Autodesk Inventor part; units mm, degrees
(part 2 of 3)
  line L290 (55.8844, 21.002) -> (55.8694, 21.0241) construction
  line L291 (55.8694, 21.0241) -> (55.8552, 21.0458) construction
  spline S93 degree 3 poles (55.8552, 21.0458) (55.8532, 21.0498) (55.8502, 21.0528) (55.8482, 21.0569) knots 0 0 0 0 1 1 1 1
  line L292 (55.8552, 21.0458) -> (55.8532, 21.0498) construction
  line L293 (55.8532, 21.0498) -> (55.8502, 21.0528) construction
  line L294 (55.8502, 21.0528) -> (55.8482, 21.0569) construction
  spline S94 degree 3 poles (55.8482, 21.0569) (55.8363, 21.0778) (55.8253, 21.0987) (55.8154, 21.1204) knots 0 0 0 0 1 1 1 1
  line L295 (55.8482, 21.0569) -> (55.8363, 21.0778) construction
  line L296 (55.8363, 21.0778) -> (55.8253, 21.0987) construction
  line L297 (55.8253, 21.0987) -> (55.8154, 21.1204) construction
  spline S95 degree 3 poles (55.8154, 21.1204) (55.8134, 21.1244) (55.8114, 21.1274) (55.8084, 21.1314) knots 0 0 0 0 1 1 1 1
  line L298 (55.8154, 21.1204) -> (55.8134, 21.1244) construction
  line L299 (55.8134, 21.1244) -> (55.8114, 21.1274) construction
  line L300 (55.8114, 21.1274) -> (55.8084, 21.1314) construction
  spline S96 degree 3 poles (55.8084, 21.1314) (55.7984, 21.1563) (55.7887, 21.1827) (55.782, 21.2079) knots 0 0 0 0 1 1 1 1
  line L301 (55.8084, 21.1314) -> (55.7984, 21.1563) construction
  line L302 (55.7984, 21.1563) -> (55.7887, 21.1827) construction
  line L303 (55.7887, 21.1827) -> (55.782, 21.2079) construction
  spline S97 degree 3 poles (55.782, 21.2079) (55.781, 21.2109) (55.78, 21.2149) (55.779, 21.2182) knots 0 0 0 0 1 1 1 1
  line L304 (55.782, 21.2079) -> (55.781, 21.2109) construction
  line L305 (55.781, 21.2109) -> (55.78, 21.2149) construction
  line L306 (55.78, 21.2149) -> (55.779, 21.2182) construction
  spline S98 degree 3 poles (55.779, 21.2182) (55.773, 21.2411) (55.7679, 21.264) (55.7652, 21.2865) knots 0 0 0 0 1 1 1 1
  line L307 (55.779, 21.2182) -> (55.773, 21.2411) construction
  line L308 (55.773, 21.2411) -> (55.7679, 21.264) construction
  line L309 (55.7679, 21.264) -> (55.7652, 21.2865) construction
  spline S99 degree 3 poles (55.7652, 21.2865) (55.7642, 21.2935) (55.7632, 21.2999) (55.7612, 21.3058) knots 0 0 0 0 1 1 1 1
  line L310 (55.7652, 21.2865) -> (55.7642, 21.2935) construction
  line L311 (55.7642, 21.2935) -> (55.7632, 21.2999) construction
  line L312 (55.7632, 21.2999) -> (55.7612, 21.3058) construction
  spline S100 degree 3 poles (55.7612, 21.3058) (55.7582, 21.333) (55.7552, 21.3595) (55.7552, 21.3863) knots 0 0 0 0 1 1 1 1
  line L313 (55.7612, 21.3058) -> (55.7582, 21.333) construction
  line L314 (55.7582, 21.333) -> (55.7552, 21.3595) construction
  line L315 (55.7552, 21.3595) -> (55.7552, 21.3863) construction
  spline S101 degree 3 poles (55.7552, 21.3863) (54.9688, 22.0101) (54.9511, 22.0101) (54.9511, 22.0101) knots 0 0 0 0 1 1 1 1
  line L316 (55.7552, 21.3863) -> (54.9688, 22.0101) construction
  line L317 (54.9688, 22.0101) -> (54.9511, 22.0101) construction
  line L318 (54.9511, 22.0101) -> (54.9511, 22.0101) construction
  line L319 (56.1953, 20.7863) -> (56.1903, 20.7883)
  spline S102 degree 3 poles (56.3621, 22.0101) (56.3747, 22.0101) (56.3877, 22.0101) (56.4012, 22.0097) knots 0 0 0 0 1 1 1 1
  line L320 (56.3621, 22.0101) -> (56.3747, 22.0101) construction
  line L321 (56.3747, 22.0101) -> (56.3877, 22.0101) construction
  line L322 (56.3877, 22.0101) -> (56.4012, 22.0097) construction
  spline S103 degree 3 poles (56.4012, 22.0097) (57.2626, 21.9765) (57.984, 20.9159) (58.8359, 20.7624) knots 0 0 0 0 1 1 1 1
  line L323 (56.4012, 22.0097) -> (57.2626, 21.9765) construction
  line L324 (57.2626, 21.9765) -> (57.984, 20.9159) construction
  line L325 (57.984, 20.9159) -> (58.8359, 20.7624) construction
  spline S104 degree 3 poles (58.8359, 20.7624) (58.5092, 20.7624) (57.8822, 20.5998) (56.9505, 21.2379) knots 0 0 0 0 1 1 1 1
  line L326 (58.8359, 20.7624) -> (58.5092, 20.7624) construction
  line L327 (58.5092, 20.7624) -> (57.8822, 20.5998) construction
  line L328 (57.8822, 20.5998) -> (56.9505, 21.2379) construction
  line L329 (54.9511, 22.0101) -> (56.3621, 22.0101)
  spline S105 degree 3 poles (56.3625, 21.7778) (56.3625, 21.7776) (56.3136, 21.6503) (56.2426, 21.554) knots 0 0 0 0 1 1 1 1
  line L330 (56.3625, 21.7778) -> (56.3625, 21.7778) construction
  line L331 (56.3625, 21.7778) -> (56.3136, 21.6503) construction
  line L332 (56.3136, 21.6503) -> (56.2426, 21.554) construction
  spline S106 degree 3 poles (56.2426, 21.554) (56.2055, 21.5027) (56.1601, 21.4546) (56.1601, 21.3863) knots 0 0 0 0 1 1 1 1
  line L333 (56.2426, 21.554) -> (56.2055, 21.5027) construction
  line L334 (56.2055, 21.5027) -> (56.1601, 21.4546) construction
  line L335 (56.1601, 21.4546) -> (56.1601, 21.3863) construction
  spline S107 degree 3 poles (56.1601, 21.3863) (56.1601, 21.318) (56.2047, 21.2699) (56.2422, 21.219) knots 0 0 0 0 1 1 1 1
  line L336 (56.1601, 21.3863) -> (56.1601, 21.318) construction
  line L337 (56.1601, 21.318) -> (56.2047, 21.2699) construction
  line L338 (56.2047, 21.2699) -> (56.2422, 21.219) construction
  spline S108 degree 3 poles (56.2422, 21.219) (56.3128, 21.1215) (56.3625, 20.9946) (56.3625, 20.9945) knots 0 0 0 0 1 1 1 1
  line L339 (56.2422, 21.219) -> (56.3128, 21.1215) construction
  line L340 (56.3128, 21.1215) -> (56.3625, 20.9945) construction
  line L341 (56.3625, 20.9945) -> (56.3625, 20.9945) construction
  spline S109 degree 3 poles (56.3625, 20.9945) (56.3626, 20.9946) (56.411, 21.1216) (56.4821, 21.2186) knots 0 0 0 0 1 1 1 1
  line L342 (56.3625, 20.9945) -> (56.3625, 20.9945) construction
  line L343 (56.3625, 20.9945) -> (56.411, 21.1216) construction
  line L344 (56.411, 21.1216) -> (56.4821, 21.2186) construction
  spline S110 degree 3 poles (56.4821, 21.2186) (56.5192, 21.2695) (56.5642, 21.3176) (56.5642, 21.3863) knots 0 0 0 0 1 1 1 1
  line L345 (56.4821, 21.2186) -> (56.5192, 21.2695) construction
  line L346 (56.5192, 21.2695) -> (56.5642, 21.3176) construction
  line L347 (56.5642, 21.3176) -> (56.5642, 21.3863) construction
  spline S111 degree 3 poles (56.5642, 21.3863) (56.5642, 21.455) (56.52, 21.5023) (56.4825, 21.5532) knots 0 0 0 0 1 1 1 1
  line L348 (56.5642, 21.3863) -> (56.5642, 21.455) construction
  line L349 (56.5642, 21.455) -> (56.52, 21.5023) construction
  line L350 (56.52, 21.5023) -> (56.4825, 21.5532) construction
  spline S112 degree 3 poles (56.4825, 21.5532) (56.4119, 21.6503) (56.3625, 21.7778) (56.3625, 21.7778) knots 0 0 0 0 1 1 1 1
  line L351 (56.4825, 21.5532) -> (56.4119, 21.6503) construction
  line L352 (56.4119, 21.6503) -> (56.3625, 21.7778) construction
  line L353 (56.3625, 21.7778) -> (56.3625, 21.7778) construction
  line L354 (56.9505, 21.2379) -> (56.9513, 21.2376)
  spline S113 degree 3 poles (56.4825, 21.5532) (56.4119, 21.6503) (56.3626, 21.7776) (56.3625, 21.7778) knots 0 0 0 0 1 1 1 1
  line L355 (56.4825, 21.5532) -> (56.4119, 21.6503) construction
  line L356 (56.4119, 21.6503) -> (56.3625, 21.7778) construction
  line L357 (56.3625, 21.7778) -> (56.3625, 21.7778) construction
  spline S114 degree 3 poles (56.3625, 21.7778) (56.3625, 21.7776) (56.3136, 21.6503) (56.2426, 21.554) knots 0 0 0 0 1 1 1 1
  line L358 (56.3625, 21.7778) -> (56.3625, 21.7778) construction
  line L359 (56.3625, 21.7778) -> (56.3136, 21.6503) construction
  line L360 (56.3136, 21.6503) -> (56.2426, 21.554) construction
  spline S115 degree 3 poles (56.2426, 21.554) (56.2055, 21.5027) (56.1601, 21.4546) (56.1601, 21.3863) knots 0 0 0 0 1 1 1 1
  line L361 (56.2426, 21.554) -> (56.2055, 21.5027) construction
  line L362 (56.2055, 21.5027) -> (56.1601, 21.4546) construction
  line L363 (56.1601, 21.4546) -> (56.1601, 21.3863) construction
  spline S116 degree 3 poles (56.1601, 21.3863) (56.1601, 21.318) (56.2047, 21.2699) (56.2422, 21.219) knots 0 0 0 0 1 1 1 1
  line L364 (56.1601, 21.3863) -> (56.1601, 21.318) construction
  line L365 (56.1601, 21.318) -> (56.2047, 21.2699) construction
  line L366 (56.2047, 21.2699) -> (56.2422, 21.219) construction
  spline S117 degree 3 poles (56.2422, 21.219) (56.3128, 21.1215) (56.3625, 20.9946) (56.3625, 20.9945) knots 0 0 0 0 1 1 1 1
  line L367 (56.2422, 21.219) -> (56.3128, 21.1215) construction
  line L368 (56.3128, 21.1215) -> (56.3625, 20.9945) construction
  line L369 (56.3625, 20.9945) -> (56.3625, 20.9945) construction
  spline S118 degree 3 poles (56.3625, 20.9945) (56.3626, 20.9946) (56.411, 21.1216) (56.4821, 21.2186) knots 0 0 0 0 1 1 1 1
  line L370 (56.3625, 20.9945) -> (56.3625, 20.9945) construction
  line L371 (56.3625, 20.9945) -> (56.411, 21.1216) construction
  line L372 (56.411, 21.1216) -> (56.4821, 21.2186) construction
  spline S119 degree 3 poles (56.4821, 21.2186) (56.5192, 21.2695) (56.5642, 21.3176) (56.5642, 21.3863) knots 0 0 0 0 1 1 1 1
  line L373 (56.4821, 21.2186) -> (56.5192, 21.2695) construction
  line L374 (56.5192, 21.2695) -> (56.5642, 21.3176) construction
  line L375 (56.5642, 21.3176) -> (56.5642, 21.3863) construction
  spline S120 degree 3 poles (56.5642, 21.3863) (56.5642, 21.455) (56.52, 21.5023) (56.4825, 21.5532) knots 0 0 0 0 1 1 1 1
  line L376 (56.5642, 21.3863) -> (56.5642, 21.455) construction
  line L377 (56.5642, 21.455) -> (56.52, 21.5023) construction
  line L378 (56.52, 21.5023) -> (56.4825, 21.5532) construction
  spline S121 degree 3 poles (62.9834, 11.6734) (62.6228, 13.9494) (60.8593, 15.3143) (55.8176, 16.2629) knots 0 0 0 0 1 1 1 1
  line L379 (62.9834, 11.6734) -> (62.6228, 13.9494) construction
  line L380 (62.6228, 13.9494) -> (60.8593, 15.3143) construction
  line L381 (60.8593, 15.3143) -> (55.8176, 16.2629) construction
  spline S122 degree 3 poles (55.8176, 16.2629) (54.8047, 16.4322) (54.6007, 17.116) (54.9542, 17.6791) knots 0 0 0 0 1 1 1 1
  line L382 (55.8176, 16.2629) -> (54.8047, 16.4322) construction
  line L383 (54.8047, 16.4322) -> (54.6007, 17.116) construction
  line L384 (54.6007, 17.116) -> (54.9542, 17.6791) construction
  spline S123 degree 3 poles (54.9542, 17.6791) (54.5048, 17.9459) (54.1315, 18.2363) (53.8782, 18.7418) knots 0 0 0 0 1 1 1 1
  line L385 (54.9542, 17.6791) -> (54.5048, 17.9459) construction
  line L386 (54.5048, 17.9459) -> (54.1315, 18.2363) construction
  line L387 (54.1315, 18.2363) -> (53.8782, 18.7418) construction
  spline S124 degree 3 poles (53.8782, 18.7418) (52.7216, 17.2451) (52.3416, 14.941) (53.1048, 13.0623) knots 0 0 0 0 1 1 1 1
  line L388 (53.8782, 18.7418) -> (52.7216, 17.2451) construction
  line L389 (52.7216, 17.2451) -> (52.3416, 14.941) construction
  line L390 (52.3416, 14.941) -> (53.1048, 13.0623) construction
  spline S125 degree 3 poles (53.1048, 13.0623) (53.1348, 13.9518) (53.525, 14.653) (54.1374, 14.9501) knots 0 0 0 0 1 1 1 1
  line L391 (53.1048, 13.0623) -> (53.1348, 13.9518) construction
  line L392 (53.1348, 13.9518) -> (53.525, 14.653) construction
  line L393 (53.525, 14.653) -> (54.1374, 14.9501) construction
  spline S126 degree 3 poles (54.1374, 14.9501) (55.0797, 15.4074) (56.4442, 15.1123) (56.5535, 14.9331) knots 0 0 0 0 1 1 1 1
  line L394 (54.1374, 14.9501) -> (55.0797, 15.4074) construction
  line L395 (55.0797, 15.4074) -> (56.4442, 15.1123) construction
  line L396 (56.4442, 15.1123) -> (56.5535, 14.9331) construction
  spline S127 degree 3 poles (56.5535, 14.9331) (55.8089, 14.8514) (55.204, 14.9371) (54.4294, 14.4249) knots 0 0 0 0 1 1 1 1
  line L397 (56.5535, 14.9331) -> (55.8089, 14.8514) construction
  line L398 (55.8089, 14.8514) -> (55.204, 14.9371) construction
  line L399 (55.204, 14.9371) -> (54.4294, 14.4249) construction
  spline S128 degree 3 poles (54.4294, 14.4249) (52.6506, 12.7652) (54.459, 11.7728) (54.7214, 11.0889) knots 0 0 0 0 1 1 1 1
  line L400 (54.4294, 14.4249) -> (52.6506, 12.7652) construction
  line L401 (52.6506, 12.7652) -> (54.459, 11.7728) construction
  line L402 (54.459, 11.7728) -> (54.7214, 11.0889) construction
  spline S129 degree 3 poles (51.5856, 11.3809) (51.0442, 10.6983) (50.6141, 10.0602) (50.4077, 9.5121) knots 0 0 0 0 1 1 1 1
  line L403 (51.5856, 11.3809) -> (51.0442, 10.6983) construction
  line L404 (51.0442, 10.6983) -> (50.6141, 10.0602) construction
  line L405 (50.6141, 10.0602) -> (50.4077, 9.5121) construction
  spline S130 degree 3 poles (50.4077, 9.5121) (50.5142, 8.7466) (50.8303, 8.2471) (51.3737, 8.032) knots 0 0 0 0 1 1 1 1
  line L406 (50.4077, 9.5121) -> (50.5142, 8.7466) construction
  line L407 (50.5142, 8.7466) -> (50.8303, 8.2471) construction
  line L408 (50.8303, 8.2471) -> (51.3737, 8.032) construction
  line L409 (54.7214, 11.0889) -> (51.5856, 11.3809)
  spline S131 degree 3 poles (51.4565, 8.4105) (51.2667, 8.7786) (51.1629, 9.1022) (51.1764, 9.3638) knots 0 0 0 0 1 1 1 1
  line L410 (51.4565, 8.4105) -> (51.2667, 8.7786) construction
  line L411 (51.2667, 8.7786) -> (51.1629, 9.1022) construction
  line L412 (51.1629, 9.1022) -> (51.1764, 9.3638) construction
  spline S132 degree 3 poles (51.1764, 9.3638) (51.3401, 9.7774) (51.6163, 10.1601) (51.9916, 10.5156) knots 0 0 0 0 1 1 1 1
  line L413 (51.1764, 9.3638) -> (51.3401, 9.7774) construction
  line L414 (51.3401, 9.7774) -> (51.6163, 10.1601) construction
  line L415 (51.6163, 10.1601) -> (51.9916, 10.5156) construction
  spline S133 degree 3 poles (51.9916, 10.5156) (52.9611, 10.1356) (54.0131, 9.8022) (55.1535, 9.5173) knots 0 0 0 0 1 1 1 1
  line L416 (51.9916, 10.5156) -> (52.9611, 10.1356) construction
  line L417 (52.9611, 10.1356) -> (54.0131, 9.8022) construction
  line L418 (54.0131, 9.8022) -> (55.1535, 9.5173) construction
  line L419 (51.3737, 8.032) -> (51.9435, 7.9914)
  line L420 (51.9435, 7.9914) -> (51.4565, 8.4105)
  spline S134 degree 3 poles (55.9166, 9.8571) (56.1155, 9.9518) (56.2978, 10.0437) (56.471, 10.1345) knots 0 0 0 0 1 1 1 1
  line L421 (55.9166, 9.8571) -> (56.1155, 9.9518) construction
  line L422 (56.1155, 9.9518) -> (56.2978, 10.0437) construction
  line L423 (56.2978, 10.0437) -> (56.471, 10.1345) construction
  line L424 (55.1535, 9.5173) -> (55.4226, 9.6373)
  line L425 (55.4226, 9.6373) -> (55.9166, 9.8571)
  spline S135 degree 3 poles (55.5457, 12.5088) (55.419, 12.7992) (55.3756, 13.0442) (55.6025, 13.1393) knots 0 0 0 0 1 1 1 1
  line L426 (55.5457, 12.5088) -> (55.419, 12.7992) construction
  line L427 (55.419, 12.7992) -> (55.3756, 13.0442) construction
  line L428 (55.3756, 13.0442) -> (55.6025, 13.1393) construction
  spline S136 degree 3 poles (55.6025, 13.1393) (56.2031, 13.1463) (56.9923, 12.9038) (57.0451, 12.8868) knots 0 0 0 0 1 1 1 1
  line L429 (55.6025, 13.1393) -> (56.2031, 13.1463) construction
  line L430 (56.2031, 13.1463) -> (56.9923, 12.9038) construction
  line L431 (56.9923, 12.9038) -> (57.0451, 12.8868) construction
  spline S137 degree 3 poles (57.0451, 12.8868) (57.0119, 12.8928) (56.6687, 12.9484) (56.0847, 12.7491) knots 0 0 0 0 1 1 1 1
  line L432 (57.0451, 12.8868) -> (57.0119, 12.8928) construction
  line L433 (57.0119, 12.8928) -> (56.6687, 12.9484) construction
  line L434 (56.6687, 12.9484) -> (56.0847, 12.7491) construction
  line L435 (56.471, 10.1345) -> (56.4552, 10.1728)
  line L436 (56.4552, 10.1728) -> (55.5457, 12.5088)
  spline S138 degree 3 poles (57.2353, 10.5733) (58.8015, 11.5763) (58.8832, 12.3995) (58.7486, 13.2656) knots 0 0 0 0 1 1 1 1
  line L437 (57.2353, 10.5733) -> (58.8015, 11.5763) construction
  line L438 (58.8015, 11.5763) -> (58.8832, 12.3995) construction
  line L439 (58.8832, 12.3995) -> (58.7486, 13.2656) construction
  spline S139 degree 3 poles (58.7486, 13.2656) (58.6819, 13.6945) (58.5655, 14.1144) (58.4025, 14.5149) knots 0 0 0 0 1 1 1 1
  line L440 (58.7486, 13.2656) -> (58.6819, 13.6945) construction
  line L441 (58.6819, 13.6945) -> (58.5655, 14.1144) construction
  line L442 (58.5655, 14.1144) -> (58.4025, 14.5149) construction
  spline S140 degree 3 poles (58.4025, 14.5149) (58.8883, 14.3949) (59.3393, 14.1554) (59.7154, 13.8161) knots 0 0 0 0 1 1 1 1
  line L443 (58.4025, 14.5149) -> (58.8883, 14.3949) construction
  line L444 (58.8883, 14.3949) -> (59.3393, 14.1554) construction
  line L445 (59.3393, 14.1554) -> (59.7154, 13.8161) construction
  spline S141 degree 3 poles (59.7154, 13.8161) (61.8793, 11.8644) (63.5682, 4.8248) (54.0229, 2.8183) knots 0 0 0 0 1 1 1 1
  line L446 (59.7154, 13.8161) -> (61.8793, 11.8644) construction
  line L447 (61.8793, 11.8644) -> (63.5682, 4.8248) construction
  line L448 (63.5682, 4.8248) -> (54.0229, 2.8183) construction
  line L449 (56.0847, 12.7491) -> (57.2353, 10.5733)
  spline S142 degree 3 poles (54.0299, 2.8183) (58.7114, 3.0811) (63.9958, 5.2928) (62.9833, 11.6734) knots 0 0 0 0 1 1 1 1
  line L450 (54.0299, 2.8183) -> (58.7114, 3.0811) construction
  line L451 (58.7114, 3.0811) -> (63.9958, 5.2928) construction
  line L452 (63.9958, 5.2928) -> (62.9833, 11.6734) construction
  line L453 (54.0229, 2.8183) -> (54.0299, 2.8183)
  line L454 (62.9833, 11.6734) -> (62.9834, 11.6734)
  point P0 (0, 0)
  constraints: 52 end point, 429 other
sketch "Szkic14" plane through (0, 0, 2.5) normal (0, 0, 1) x (1, 0, 0)
  line L0 (-6.6512, 10.9422) -> (-6.5928, 10.8137) construction
  line L1 (-6.5928, 10.8137) -> (-6.4673, 10.6328) construction
  line L2 (-6.4673, 10.6328) -> (-6.3389, 10.4489) construction
  line L3 (-6.3389, 10.4489) -> (-6.0849, 10.1628) construction
  line L4 (-6.0849, 10.1628) -> (-5.8893, 9.9935) construction
  line L5 (-5.8893, 9.9935) -> (-5.6704, 9.8271) construction
  line L6 (-5.6704, 9.8271) -> (-5.4544, 9.687) construction
  line L7 (-5.4544, 9.687) -> (-5.2589, 9.5674) construction
  spline S0 degree 4 poles (-6.6512, 10.9422) (-6.5928, 10.8137) (-6.4673, 10.6328) (-6.3389, 10.4489) (-6.0849, 10.1628) (-5.8893, 9.9935) (-5.6704, 9.8271) (-5.4544, 9.687) (-5.2589, 9.5674) knots 1 1 1 1 1 2 3 4 5 6 6 6 6 6
  line L8 (-5.2589, 9.5674) -> (-5.4035, 9.331) construction
  line L9 (-5.4035, 9.331) -> (-5.4544, 9.0682) construction
  line L10 (-5.4544, 9.0682) -> (-5.4544, 8.9077) construction
  line L11 (-5.4544, 8.9077) -> (-5.4544, 8.7325) construction
  line L12 (-5.4544, 8.7325) -> (-5.4106, 8.5574) construction
  line L13 (-5.4106, 8.5574) -> (-5.3378, 8.3971) construction
  line L14 (-5.3378, 8.3971) -> (-5.2384, 8.2538) construction
  line L15 (-5.2384, 8.2538) -> (-5.0652, 8.1039) construction
  line L16 (-5.0652, 8.1039) -> (-4.9181, 7.9921) construction
  line L17 (-4.9181, 7.9921) -> (-4.7393, 7.8984) construction
  line L18 (-4.7393, 7.8984) -> (-4.596, 7.8481) construction
  line L19 (-4.596, 7.8481) -> (-4.3639, 7.7777) construction
  line L20 (-4.3639, 7.7777) -> (-4.0614, 7.7125) construction
  line L21 (-4.0614, 7.7125) -> (-3.7401, 7.6548) construction
  line L22 (-3.7401, 7.6548) -> (-3.2763, 7.5488) construction
  line L23 (-3.2763, 7.5488) -> (-2.8258, 7.4561) construction
  spline S1 degree 4 poles (-5.2589, 9.5674) (-5.4035, 9.331) (-5.4544, 9.0682) (-5.4544, 8.9077) (-5.4544, 8.7325) (-5.4106, 8.5574) (-5.3378, 8.3971) (-5.2384, 8.2538) (-5.0652, 8.1039) (-4.9181, 7.9921) (-4.7393, 7.8984) (-4.596, 7.8481) (-4.3639, 7.7777) (-4.0614, 7.7125) (-3.7401, 7.6548) (-3.2763, 7.5488) (-2.8258, 7.4561) knots 1 1 1 1 1 2 3 4 5 6 7 8 9 10 11 12 13 14 14 14 14 14
  line L24 (-2.8258, 7.4561) -> (-2.2142, 7.3144) construction
  line L25 (-2.2142, 7.3144) -> (-1.5745, 7.1703) construction
  line L26 (-1.5745, 7.1703) -> (-0.9584, 6.9834) construction
  line L27 (-0.9584, 6.9834) -> (-0.2587, 6.7712) construction
  line L28 (-0.2587, 6.7712) -> (0.4179, 6.5333) construction
  line L29 (0.4179, 6.5333) -> (1.2289, 6.2149) construction
  line L30 (1.2289, 6.2149) -> (1.8914, 5.9102) construction
  line L31 (1.8914, 5.9102) -> (2.8245, 5.3392) construction
  line L32 (2.8245, 5.3392) -> (3.3345, 4.9516) construction
  line L33 (3.3345, 4.9516) -> (3.839, 4.4666) construction
  line L34 (3.839, 4.4666) -> (4.1432, 4.1239) construction
  line L35 (4.1432, 4.1239) -> (4.4557, 3.6733) construction
  line L36 (4.4557, 3.6733) -> (4.6713, 3.2438) construction
  line L37 (4.6713, 3.2438) -> (4.8704, 2.8057) construction
  line L38 (4.8704, 2.8057) -> (4.945, 2.5074) construction
  line L39 (4.945, 2.5074) -> (5.0688, 2.0124) construction
  line L40 (5.0688, 2.0124) -> (5.1432, 1.5744) construction
  line L41 (5.1432, 1.5744) -> (5.1888, 0.9732) construction
  line L42 (5.1888, 0.9732) -> (5.2151, 0.3807) construction
  line L43 (5.2151, 0.3807) -> (5.2602, -0.5324) construction
  line L44 (5.2602, -0.5324) -> (5.1507, -1.5377) construction
  line L45 (5.1507, -1.5377) -> (4.9589, -2.5271) construction
  line L46 (4.9589, -2.5271) -> (4.707, -3.3577) construction
  line L47 (4.707, -3.3577) -> (4.6129, -3.6252) construction
  line L48 (4.6129, -3.6252) -> (4.4152, -4.0747) construction
  line L49 (4.4152, -4.0747) -> (3.746, -5.2202) construction
  line L50 (3.746, -5.2202) -> (3.0018, -6.0798) construction
  line L51 (3.0018, -6.0798) -> (2.3815, -6.6305) construction
  line L52 (2.3815, -6.6305) -> (1.6684, -7.2033) construction
  line L53 (1.6684, -7.2033) -> (0.6461, -7.8274) construction
  line L54 (0.6461, -7.8274) -> (-0.713, -8.472) construction
  line L55 (-0.713, -8.472) -> (-2.0638, -8.9236) construction
  line L56 (-2.0638, -8.9236) -> (-3.5466, -9.2943) construction
  line L57 (-3.5466, -9.2943) -> (-5.0652, -9.5408) construction
  line L58 (-5.0652, -9.5408) -> (-6.4673, -9.6692) construction
  spline S2 degree 4 poles (-2.8258, 7.4561) (-2.2142, 7.3144) (-1.5745, 7.1703) (-0.9584, 6.9834) (-0.2587, 6.7712) (0.4179, 6.5333) (1.2289, 6.2149) (1.8914, 5.9102) (2.8245, 5.3392) (3.3345, 4.9516) (3.839, 4.4666) (4.1432, 4.1239) (4.4557, 3.6733) (4.6713, 3.2438) (4.8704, 2.8057) (4.945, 2.5074) (5.0688, 2.0124) (5.1432, 1.5744) (5.1888, 0.9732) (5.2151, 0.3807) (5.2602, -0.5324) (5.1507, -1.5377) (4.9589, -2.5271) (4.707, -3.3577) (4.6129, -3.6252) (4.4152, -4.0747) (3.746, -5.2202) (3.0018, -6.0798) (2.3815, -6.6305) (1.6684, -7.2033) (0.6461, -7.8274) (-0.713, -8.472) (-2.0638, -8.9236) (-3.5466, -9.2943) (-5.0652, -9.5408) (-6.4673, -9.6692) knots 1 1 1 1 1 2 3 4 5 6 7 8 9 10 11 12 13 14 15 16 17 18 19 20 21 22 23 24 25 26 27 28 29 30 31 32 33 33 33 33 33
  line L59 (-6.4673, -9.6692) -> (-4.596, -9.174) construction
  line L60 (-4.596, -9.174) -> (-3.6929, -8.872) construction
  line L61 (-3.6929, -8.872) -> (-2.1422, -8.2833) construction
  line L62 (-2.1422, -8.2833) -> (-1.296, -7.901) construction
  line L63 (-1.296, -7.901) -> (-0.6086, -7.3619) construction
  line L64 (-0.6086, -7.3619) -> (0.1327, -6.8478) construction
  line L65 (0.1327, -6.8478) -> (0.6779, -6.2808) construction
  line L66 (0.6779, -6.2808) -> (1.3083, -5.7211) construction
  line L67 (1.3083, -5.7211) -> (1.8469, -5.0124) construction
  line L68 (1.8469, -5.0124) -> (2.3815, -4.2056) construction
  line L69 (2.3815, -4.2056) -> (2.5915, -3.6252) construction
  line L70 (2.5915, -3.6252) -> (2.7867, -2.9832) construction
  line L71 (2.7867, -2.9832) -> (2.8933, -2.4331) construction
  line L72 (2.8933, -2.4331) -> (2.9439, -2.2891) construction
  line L73 (2.9439, -2.2891) -> (3.0251, -1.8703) construction
  line L74 (3.0251, -1.8703) -> (3.0795, -1.3802) construction
  line L75 (3.0795, -1.3802) -> (3.0795, -0.9391) construction
  line L76 (3.0795, -0.9391) -> (3.0444, -0.4767) construction
  line L77 (3.0444, -0.4767) -> (3.0018, 0.0093) construction
  line L78 (3.0018, 0.0093) -> (2.9748, 0.3807) construction
  line L79 (2.9748, 0.3807) -> (2.902, 0.7996) construction
  line L80 (2.902, 0.7996) -> (2.8245, 1.096) construction
  line L81 (2.8245, 1.096) -> (2.6916, 1.5744) construction
  line L82 (2.6916, 1.5744) -> (2.5274, 2.0615) construction
  line L83 (2.5274, 2.0615) -> (2.358, 2.4623) construction
  line L84 (2.358, 2.4623) -> (2.1656, 2.8856) construction
  line L85 (2.1656, 2.8856) -> (1.8914, 3.3203) construction
  line L86 (1.8914, 3.3203) -> (1.5602, 3.796) construction
  line L87 (1.5602, 3.796) -> (1.1327, 4.2607) construction
  line L88 (1.1327, 4.2607) -> (0.6123, 4.7937) construction
  line L89 (0.6123, 4.7937) -> (-0.1776, 5.2552) construction
  line L90 (-0.1776, 5.2552) -> (-0.7923, 5.4713) construction
  spline S3 degree 4 poles (-6.4673, -9.6692) (-4.596, -9.174) (-3.6929, -8.872) (-2.1422, -8.2833) (-1.296, -7.901) (-0.6086, -7.3619) (0.1327, -6.8478) (0.6779, -6.2808) (1.3083, -5.7211) (1.8469, -5.0124) (2.3815, -4.2056) (2.5915, -3.6252) (2.7867, -2.9832) (2.8933, -2.4331) (2.9439, -2.2891) (3.0251, -1.8703) (3.0795, -1.3802) (3.0795, -0.9391) (3.0444, -0.4767) (3.0018, 0.0093) (2.9748, 0.3807) (2.902, 0.7996) (2.8245, 1.096) (2.6916, 1.5744) (2.5274, 2.0615) (2.358, 2.4623) (2.1656, 2.8856) (1.8914, 3.3203) (1.5602, 3.796) (1.1327, 4.2607) (0.6123, 4.7937) (-0.1776, 5.2552) (-0.7923, 5.4713) knots 1 1 1 1 1 2 3 4 5 6 7 8 9 10 11 12 13 14 15 16 17 18 19 20 21 22 23 24 25 26 27 28 29 30 30 30 30 30
  line L91 (-0.7923, 5.4713) -> (-0.4849, 4.5272) construction
  line L92 (-0.4849, 4.5272) -> (-0.4074, 4.1857) construction
  line L93 (-0.4074, 4.1857) -> (-0.3088, 3.605) construction
  line L94 (-0.3088, 3.605) -> (-0.2587, 3.1864) construction
  line L95 (-0.2587, 3.1864) -> (-0.3231, 2.5956) construction
  line L96 (-0.3231, 2.5956) -> (-0.6086, 2.0124) construction
  line L97 (-0.6086, 2.0124) -> (-0.9875, 1.4524) construction
  line L98 (-0.9875, 1.4524) -> (-1.296, 1.0568) construction
  line L99 (-1.296, 1.0568) -> (-1.7784, 0.7017) construction
  line L100 (-1.7784, 0.7017) -> (-2.309, 0.344) construction
  spline S4 degree 4 poles (-0.7923, 5.4713) (-0.4849, 4.5272) (-0.4074, 4.1857) (-0.3088, 3.605) (-0.2587, 3.1864) (-0.3231, 2.5956) (-0.6086, 2.0124) (-0.9875, 1.4524) (-1.296, 1.0568) (-1.7784, 0.7017) (-2.309, 0.344) knots 1 1 1 1 1 2 3 4 5 6 7 8 8 8 8 8
  line L101 (-2.309, 0.344) -> (-2.5669, 0.9223) construction
  line L102 (-2.5669, 0.9223) -> (-2.9657, 1.6305) construction
  line L103 (-2.9657, 1.6305) -> (-3.1735, 2.0877) construction
  line L104 (-3.1735, 2.0877) -> (-3.4271, 2.6566) construction
  line L105 (-3.4271, 2.6566) -> (-3.8071, 3.1864) construction
  spline S5 degree 4 poles (-2.309, 0.344) (-2.5669, 0.9223) (-2.9657, 1.6305) (-3.1735, 2.0877) (-3.4271, 2.6566) (-3.8071, 3.1864) knots 1 1 1 1 1 2 3 3 3 3 3
  line L106 (-3.8071, 3.1864) -> (-3.5082, 3.2675) construction
  line L107 (-3.5082, 3.2675) -> (-3.101, 3.3757) construction
  line L108 (-3.101, 3.3757) -> (-2.5516, 3.3626) construction
  spline S6 degree 3 poles (-3.8071, 3.1864) (-3.5082, 3.2675) (-3.101, 3.3757) (-2.5516, 3.3626) knots 1 1 1 1 2 2 2 2
  line L109 (-2.5516, 3.3626) -> (-3.6577, 3.6945) construction
  line L110 (-3.6577, 3.6945) -> (-4.4013, 3.6945) construction
  spline S7 degree 2 poles (-2.5516, 3.3626) (-3.6577, 3.6945) (-4.4013, 3.6945) knots 1 1 1 2 2 2
  line L111 (-4.4013, 3.6945) -> (-4.7094, 3.5581) construction
  line L112 (-4.7094, 3.5581) -> (-4.6553, 3.2438) construction
  line L113 (-4.6553, 3.2438) -> (-4.5019, 2.891) construction
  spline S8 degree 3 poles (-4.4013, 3.6945) (-4.7094, 3.5581) (-4.6553, 3.2438) (-4.5019, 2.891) knots 1 1 1 1 2 2 2 2
  line L114 (-4.5019, 2.891) -> (-3.2936, -0.1999) construction
  spline S9 degree 1 poles (-4.5019, 2.891) (-3.2936, -0.1999) knots 1 1 2 2
  line L115 (-3.2936, -0.1999) -> (-4.9917, -1.0028) construction
  spline S10 degree 1 poles (-3.2936, -0.1999) (-4.9917, -1.0028) knots 1 1 2 2
  line L116 (-4.9917, -1.0028) -> (-6.474, -0.6289) construction
  line L117 (-6.474, -0.6289) -> (-7.8356, -0.1999) construction
  line L118 (-7.8356, -0.1999) -> (-9.0893, 0.2923) construction
  spline S11 degree 3 poles (-4.9917, -1.0028) (-6.474, -0.6289) (-7.8356, -0.1999) (-9.0893, 0.2923) knots 1 1 1 1 2 2 2 2
  line L119 (-9.0893, 0.2923) -> (-9.5782, -0.1675) construction
  line L120 (-9.5782, -0.1675) -> (-9.9324, -0.6627) construction
  line L121 (-9.9324, -0.6627) -> (-10.1402, -1.1921) construction
  spline S12 degree 3 poles (-9.0893, 0.2923) (-9.5782, -0.1675) (-9.9324, -0.6627) (-10.1402, -1.1921) knots 1 1 1 1 2 2 2 2
  line L122 (-10.1402, -1.1921) -> (-10.1643, -1.5377) construction
  line L123 (-10.1643, -1.5377) -> (-10.0286, -1.9545) construction
  line L124 (-10.0286, -1.9545) -> (-9.7859, -2.4331) construction
  spline S13 degree 3 poles (-10.1402, -1.1921) (-10.1643, -1.5377) (-10.0286, -1.9545) (-9.7859, -2.4331) knots 1 1 1 1 2 2 2 2
  line L125 (-9.7859, -2.4331) -> (-9.159, -2.9734) construction
  spline S14 degree 1 poles (-9.7859, -2.4331) (-9.159, -2.9734) knots 1 1 2 2
  line L126 (-9.159, -2.9734) -> (-9.8893, -2.9225) construction
  spline S15 degree 1 poles (-9.159, -2.9734) (-9.8893, -2.9225) knots 1 1 2 2
  line L127 (-9.8893, -2.9225) -> (-10.5931, -2.6463) construction
  line L128 (-10.5931, -2.6463) -> (-10.9937, -1.9901) construction
  line L129 (-10.9937, -1.9901) -> (-11.1401, -1.006) construction
  spline S16 degree 3 poles (-9.8893, -2.9225) (-10.5931, -2.6463) (-10.9937, -1.9901) (-11.1401, -1.006) knots 1 1 1 1 2 2 2 2
  line L130 (-11.1401, -1.006) -> (-10.8707, -0.2943) construction
  line L131 (-10.8707, -0.2943) -> (-10.3129, 0.5299) construction
  line L132 (-10.3129, 0.5299) -> (-9.6159, 1.4127) construction
  spline S17 degree 3 poles (-11.1401, -1.006) (-10.8707, -0.2943) (-10.3129, 0.5299) (-9.6159, 1.4127) knots 1 1 1 1 2 2 2 2
  line L133 (-9.6159, 1.4127) -> (-5.5569, 1.0352) construction
  spline S18 degree 1 poles (-9.6159, 1.4127) (-5.5569, 1.0352) knots 1 1 2 2
  line L134 (-5.5569, 1.0352) -> (-5.8976, 1.9192) construction
  line L135 (-5.8976, 1.9192) -> (-8.2266, 3.1864) construction
  line L136 (-8.2266, 3.1864) -> (-5.9522, 5.3392) construction
  spline S19 degree 3 poles (-5.5569, 1.0352) (-5.8976, 1.9192) (-8.2266, 3.1864) (-5.9522, 5.3392) knots 1 1 1 1 2 2 2 2
  line L137 (-5.925, 5.3649) -> (-4.934, 6.0162) construction
  line L138 (-4.934, 6.0162) -> (-4.1426, 5.9102) construction
  line L139 (-4.1426, 5.9102) -> (-3.1879, 5.9976) construction
  spline S20 degree 3 poles (-5.925, 5.3649) (-4.934, 6.0162) (-4.1426, 5.9102) (-3.1879, 5.9976) knots 1 1 1 1 2 2 2 2
  line L140 (-3.1879, 5.9976) -> (-3.3286, 6.2406) construction
  line L141 (-3.3286, 6.2406) -> (-5.0959, 6.6215) construction
  line L142 (-5.0959, 6.6215) -> (-6.3118, 6.0277) construction
  spline S21 degree 3 poles (-3.1879, 5.9976) (-3.3286, 6.2406) (-5.0959, 6.6215) (-6.3118, 6.0277) knots 1 1 1 1 2 2 2 2
  line L143 (-6.3118, 6.0277) -> (-7.1084, 5.6386) construction
  line L144 (-7.1084, 5.6386) -> (-7.6107, 4.7393) construction
  line L145 (-7.6107, 4.7393) -> (-7.6499, 3.5891) construction
  spline S22 degree 3 poles (-6.3118, 6.0277) (-7.1084, 5.6386) (-7.6107, 4.7393) (-7.6499, 3.5891) knots 1 1 1 1 2 2 2 2
  line L146 (-7.6499, 3.5891) -> (-8.6374, 6.0197) construction
  line L147 (-8.6374, 6.0197) -> (-8.1455, 9.0016) construction
  line L148 (-8.1455, 9.0016) -> (-6.6512, 10.9422) construction
  spline S23 degree 3 poles (-7.6499, 3.5891) (-8.6374, 6.0197) (-8.1455, 9.0016) (-6.6512, 10.9422) knots 1 1 1 1 2 2 2 2
  line L149 (0.3944, 2.4753) -> (0.1344, 1.2546) construction
  line L150 (0.1344, 1.2546) -> (-0.8971, 0.0624) construction
  line L151 (-0.8971, 0.0624) -> (-3.5466, -1.1921) construction
  spline S24 degree 3 poles (0.3944, 2.4753) (0.1344, 1.2546) (-0.8971, 0.0624) (-3.5466, -1.1921) knots 1 1 1 1 2 2 2 2
  line L152 (-3.5466, -1.1921) -> (-5.9451, -2.3374) construction
  line L153 (-5.9451, -2.3374) -> (-9.2943, -4.9163) construction
  line L154 (-9.2943, -4.9163) -> (-10.5452, -8.3223) construction
  spline S25 degree 3 poles (-3.5466, -1.1921) (-5.9451, -2.3374) (-9.2943, -4.9163) (-10.5452, -8.3223) knots 1 1 1 1 2 2 2 2
  line L155 (-10.5452, -8.3223) -> (-8.6452, -6.059) construction
  line L156 (-8.6452, -6.059) -> (-5.4106, -5.4167) construction
  line L157 (-5.4106, -5.4167) -> (-2.9657, -4.3118) construction
  spline S26 degree 3 poles (-10.5452, -8.3223) (-8.6452, -6.059) (-5.4106, -5.4167) (-2.9657, -4.3118) knots 1 1 1 1 2 2 2 2
  line L158 (-2.9657, -4.3118) -> (-1.5872, -3.6709) construction
  line L159 (-1.5872, -3.6709) -> (-0.4658, -2.9113) construction
  line L160 (-0.4658, -2.9113) -> (0.1531, -1.6598) construction
  spline S27 degree 3 poles (-2.9657, -4.3118) (-1.5872, -3.6709) (-0.4658, -2.9113) (0.1531, -1.6598) knots 1 1 1 1 2 2 2 2
  line L161 (0.1531, -1.6598) -> (0.6123, -0.7315) construction
  line L162 (0.6123, -0.7315) -> (0.7792, 0.5902) construction
  line L163 (0.7792, 0.5902) -> (0.3944, 2.4753) construction
  spline S28 degree 3 poles (0.1531, -1.6598) (0.6123, -0.7315) (0.7792, 0.5902) (0.3944, 2.4753) knots 1 1 1 1 2 2 2 2
  line L164 (-10.4076, -9.4348) -> (-8.846, -6.9626) construction
  line L165 (-8.846, -6.9626) -> (-5.4662, -6.2985) construction
  line L166 (-5.4662, -6.2985) -> (-2.64, -5.0124) construction
  spline S29 degree 3 poles (-10.4076, -9.4348) (-8.846, -6.9626) (-5.4662, -6.2985) (-2.64, -5.0124) knots 1 1 1 1 2 2 2 2
  line L167 (-2.64, -5.0124) -> (-1.2049, -4.3594) construction
  line L168 (-1.2049, -4.3594) -> (0.0973, -3.5037) construction
  line L169 (0.0973, -3.5037) -> (0.7792, -2.0679) construction
  spline S30 degree 3 poles (-2.64, -5.0124) (-1.2049, -4.3594) (0.0973, -3.5037) (0.7792, -2.0679) knots 1 1 1 1 2 2 2 2
  line L170 (0.7792, -2.0679) -> (1.4575, -0.7723) construction
  line L171 (1.4575, -0.7723) -> (1.5746, 0.9478) construction
  line L172 (1.5746, 0.9478) -> (0.9836, 3.3002) construction
  spline S31 degree 3 poles (0.7792, -2.0679) (1.4575, -0.7723) (1.5746, 0.9478) (0.9836, 3.3002) knots 1 1 1 1 2 2 2 2
  line L173 (0.9836, 3.3002) -> (3.1145, 0.2876) construction
  line L174 (3.1145, 0.2876) -> (4.535, -8.2093) construction
  line L175 (4.535, -8.2093) -> (-10.4076, -9.4348) construction
  spline S32 degree 3 poles (0.9836, 3.3002) (3.1145, 0.2876) (4.535, -8.2093) (-10.4076, -9.4348) knots 1 1 1 1 2 2 2 2
  line L176 (-8.4554, 3.5501) -> (-9.4517, 6.2736) construction
  line L177 (-9.4517, 6.2736) -> (-8.8433, 9.4794) construction
  line L178 (-8.8433, 9.4794) -> (-6.9806, 11.751) construction
  spline S33 degree 3 poles (-8.4554, 3.5501) (-9.4517, 6.2736) (-8.8433, 9.4794) (-6.9806, 11.751) knots 1 1 1 1 2 2 2 2
  line L179 (-6.9806, 11.751) -> (-7.1817, 12.3523) construction
  line L180 (-7.1817, 12.3523) -> (-7.2622, 12.8484) construction
  line L181 (-7.2622, 12.8484) -> (-7.2041, 12.8754) construction
  spline S34 degree 3 poles (-6.9806, 11.751) (-7.1817, 12.3523) (-7.2622, 12.8484) (-7.2041, 12.8754) knots 1 1 1 1 2 2 2 2
  line L182 (-7.2041, 12.8754) -> (-6.876, 12.3675) construction
  line L183 (-6.876, 12.3675) -> (-6.5573, 11.8558) construction
  line L184 (-6.5573, 11.8558) -> (-6.161, 11.3808) construction
  spline S35 degree 3 poles (-7.2041, 12.8754) (-6.876, 12.3675) (-6.5573, 11.8558) (-6.161, 11.3808) knots 1 1 1 1 2 2 2 2
  line L185 (-6.161, 11.3808) -> (-5.6256, 10.7423) construction
  line L186 (-5.6256, 10.7423) -> (-4.9415, 10.2089) construction
  line L187 (-4.9415, 10.2089) -> (-3.9139, 9.9917) construction
  spline S36 degree 3 poles (-6.161, 11.3808) (-5.6256, 10.7423) (-4.9415, 10.2089) (-3.9139, 9.9917) knots 1 1 1 1 2 2 2 2
  line L188 (-3.9139, 9.9917) -> (-1.4938, 10.659) construction
  line L189 (-1.4938, 10.659) -> (0.3766, 10.3417) construction
  line L190 (0.3766, 10.3417) -> (0.7325, 10.4159) construction
  spline S37 degree 3 poles (-3.9139, 9.9917) (-1.4938, 10.659) (0.3766, 10.3417) (0.7325, 10.4159) knots 1 1 1 1 2 2 2 2
  line L191 (0.7325, 10.4159) -> (0.7743, 10.4299) construction
  spline S38 degree 1 poles (0.7325, 10.4159) (0.7743, 10.4299) knots 1 1 2 2
  line L192 (0.7743, 10.4299) -> (1.3572, 10.5696) construction
  line L193 (1.3572, 10.5696) -> (1.7028, 10.8019) construction
  line L194 (1.7028, 10.8019) -> (1.9632, 11.0675) construction
  spline S39 degree 3 poles (0.7743, 10.4299) (1.3572, 10.5696) (1.7028, 10.8019) (1.9632, 11.0675) knots 1 1 1 1 2 2 2 2
  line L195 (1.9632, 11.0675) -> (1.4112, 11.4596) construction
  line L196 (1.4112, 11.4596) -> (0.6576, 11.4076) construction
  line L197 (0.6576, 11.4076) -> (-0.3268, 11.2832) construction
  spline S40 degree 3 poles (1.9632, 11.0675) (1.4112, 11.4596) (0.6576, 11.4076) (-0.3268, 11.2832) knots 1 1 1 1 2 2 2 2
  line L198 (-0.3268, 11.2832) -> (-2.8674, 10.9624) construction
  line L199 (-2.8674, 10.9624) -> (-3.5966, 11.583) construction
  line L200 (-3.5966, 11.583) -> (-4.8507, 12.8746) construction
  spline S41 degree 3 poles (-0.3268, 11.2832) (-2.8674, 10.9624) (-3.5966, 11.583) (-4.8507, 12.8746) knots 1 1 1 1 2 2 2 2
  line L201 (-4.8507, 12.8746) -> (-1.8689, 11.8753) construction
  line L202 (-1.8689, 11.8753) -> (-0.3173, 12.0747) construction
  spline S42 degree 2 poles (-4.8507, 12.8746) (-1.8689, 11.8753) (-0.3173, 12.0747) knots 1 1 1 2 2 2
  line L203 (-0.3173, 12.0747) -> (0.5689, 12.1885) construction
  line L204 (0.5689, 12.1885) -> (1.6252, 12.4242) construction
  line L205 (1.6252, 12.4242) -> (2.2144, 11.815) construction
  spline S43 degree 3 poles (-0.3173, 12.0747) (0.5689, 12.1885) (1.6252, 12.4242) (2.2144, 11.815) knots 1 1 1 1 2 2 2 2
  line L206 (2.2144, 11.815) -> (2.2933, 12.2553) construction
  spline S44 degree 1 poles (2.2144, 11.815) (2.2933, 12.2553) knots 1 1 2 2
  line L207 (2.2933, 12.2553) -> (2.1499, 14.0918) construction
  line L208 (2.1499, 14.0918) -> (-2.5759, 16.2657) construction
  line L209 (-2.5759, 16.2657) -> (-5.495, 16.2103) construction
  spline S45 degree 3 poles (2.2933, 12.2553) (2.1499, 14.0918) (-2.5759, 16.2657) (-5.495, 16.2103) knots 1 1 1 1 2 2 2 2
  line L210 (-5.495, 16.2103) -> (-7.2811, 16.1764) construction
  line L211 (-7.2811, 16.1764) -> (-8.9609, 15.5386) construction
  line L212 (-8.9609, 15.5386) -> (-10.6059, 14.1362) construction
  spline S46 degree 3 poles (-5.495, 16.2103) (-7.2811, 16.1764) (-8.9609, 15.5386) (-10.6059, 14.1362) knots 1 1 1 1 2 2 2 2
  line L213 (-10.6059, 14.1362) -> (-9.4347, 14.6049) construction
  line L214 (-9.4347, 14.6049) -> (-8.4418, 14.7262) construction
  line L215 (-8.4418, 14.7262) -> (-7.5526, 14.6511) construction
  spline S47 degree 3 poles (-10.6059, 14.1362) (-9.4347, 14.6049) (-8.4418, 14.7262) (-7.5526, 14.6511) knots 1 1 1 1 2 2 2 2
  line L216 (-7.5526, 14.6511) -> (-11.1454, 13.1841) construction
  line L217 (-11.1454, 13.1841) -> (-11.2737, 9.7093) construction
  line L218 (-11.2737, 9.7093) -> (-11.2386, 8.7565) construction
  spline S48 degree 3 poles (-7.5526, 14.6511) (-11.1454, 13.1841) (-11.2737, 9.7093) (-11.2386, 8.7565) knots 1 1 1 1 2 2 2 2
  line L219 (-11.2386, 8.7565) -> (-10.976, 10.006) construction
  line L220 (-10.976, 10.006) -> (-10.3353, 11.0675) construction
  line L221 (-10.3353, 11.0675) -> (-9.3072, 11.9348) construction
  spline S49 degree 3 poles (-11.2386, 8.7565) (-10.976, 10.006) (-10.3353, 11.0675) (-9.3072, 11.9348) knots 1 1 1 1 2 2 2 2
  line L222 (-9.3072, 11.9348) -> (-10.918, 9.2502) construction
  line L223 (-10.918, 9.2502) -> (-10.8983, 6.1367) construction
  line L224 (-10.8983, 6.1367) -> (-8.7946, 3.9068) construction
  line L225 (-8.7946, 3.9068) -> (-8.6241, 3.7285) construction
  line L226 (-8.6241, 3.7285) -> (-8.4554, 3.5501) construction
  spline S50 degree 4 poles (-9.3072, 11.9348) (-10.918, 9.2502) (-10.8983, 6.1367) (-8.7946, 3.9068) (-8.6241, 3.7285) (-8.4554, 3.5501) knots 1 1 1 1 1 2 3 3 3 3 3
  line L227 (-8.2872, 2.2556) -> (-10.084, 4.1479) construction
  spline S51 degree 1 poles (-8.2872, 2.2556) (-10.084, 4.1479) knots 1 1 2 2
  line L228 (-10.084, 4.1479) -> (-11.2771, 4.2886) construction
  spline S52 degree 1 poles (-10.084, 4.1479) (-11.2771, 4.2886) knots 1 1 2 2
  line L229 (-11.2771, 4.2886) -> (-11.8986, 3.6234) construction
  line L230 (-11.8986, 3.6234) -> (-12.4304, 2.8856) construction
  line L231 (-12.4304, 2.8856) -> (-12.9043, 2.105) construction
  spline S53 degree 3 poles (-11.2771, 4.2886) (-11.8986, 3.6234) (-12.4304, 2.8856) (-12.9043, 2.105) knots 1 1 1 1 2 2 2 2
  line L232 (-12.9043, 2.105) -> (-12.9043, 1.7648) construction
  line L233 (-12.9043, 1.7648) -> (-12.8529, 1.4217) construction
  line L234 (-12.8529, 1.4217) -> (-12.7072, 1.0737) construction
  spline S54 degree 3 poles (-12.9043, 2.105) (-12.9043, 1.7648) (-12.8529, 1.4217) (-12.7072, 1.0737) knots 1 1 1 1 2 2 2 2
  line L235 (-12.7072, 1.0737) -> (-12.4191, 0.426) construction
  line L236 (-12.4191, 0.426) -> (-12.0213, 0.0935) construction
  line L237 (-12.0213, 0.0935) -> (-11.5184, 0.0496) construction
  spline S55 degree 3 poles (-12.7072, 1.0737) (-12.4191, 0.426) (-12.0213, 0.0935) (-11.5184, 0.0496) knots 1 1 1 1 2 2 2 2
  line L238 (-11.5184, 0.0496) -> (-11.8379, 0.4444) construction
  line L239 (-11.8379, 0.4444) -> (-11.9856, 0.8243) construction
  line L240 (-11.9856, 0.8243) -> (-12.0374, 1.2029) construction
  spline S56 degree 3 poles (-11.5184, 0.0496) (-11.8379, 0.4444) (-11.9856, 0.8243) (-12.0374, 1.2029) knots 1 1 1 1 2 2 2 2
  line L241 (-12.0374, 1.2029) -> (-12.0632, 1.431) construction
  line L242 (-12.0632, 1.431) -> (-11.5386, 2.6332) construction
  line L243 (-11.5386, 2.6332) -> (-10.9727, 2.9857) construction
  spline S57 degree 3 poles (-12.0374, 1.2029) (-12.0632, 1.431) (-11.5386, 2.6332) (-10.9727, 2.9857) knots 1 1 1 1 2 2 2 2
  line L244 (-10.9727, 2.9857) -> (-10.7928, 2.9973) construction
  line L245 (-10.7928, 2.9973) -> (-9.8119, 2.6965) construction
  line L246 (-9.8119, 2.6965) -> (-8.6066, 2.3085) construction
  spline S58 degree 3 poles (-10.9727, 2.9857) (-10.7928, 2.9973) (-9.8119, 2.6965) (-8.6066, 2.3085) knots 1 1 1 1 2 2 2 2
  line L247 (-8.6066, 2.3085) -> (-8.2872, 2.2556) construction
  spline S59 degree 1 poles (-8.6066, 2.3085) (-8.2872, 2.2556) knots 1 1 2 2
  line L248 (-4.22, 14.3594) -> (-5.2384, 15.1671) construction
  line L249 (-5.2384, 15.1671) -> (-5.2608, 15.1666) construction
  spline S60 degree 2 poles (-4.22, 14.3594) (-5.2384, 15.1671) (-5.2608, 15.1666) knots 1 1 1 2 2 2
  line L250 (-5.2608, 15.1666) -> (-3.4185, 15.1666) construction
  spline S61 degree 1 poles (-5.2608, 15.1666) (-3.4185, 15.1666) knots 1 1 2 2
  line L251 (-3.4185, 15.1666) -> (-3.4019, 15.1666) construction
  line L252 (-3.4019, 15.1666) -> (-2.2715, 15.1248) construction
  line L253 (-2.2715, 15.1248) -> (-1.3354, 13.7496) construction
  line L254 (-1.3354, 13.7496) -> (-0.2343, 13.5521) construction
  spline S62 degree 4 poles (-3.4185, 15.1666) (-3.4019, 15.1666) (-2.2715, 15.1248) (-1.3354, 13.7496) (-0.2343, 13.5521) knots 1 1 1 1 1 2 2 2 2 2
  line L255 (-0.2343, 13.5521) -> (-0.6559, 13.5521) construction
  line L256 (-0.6559, 13.5521) -> (-1.4682, 13.3417) construction
  line L257 (-1.4682, 13.3417) -> (-2.673, 14.1668) construction
  spline S63 degree 3 poles (-0.2343, 13.5521) (-0.6559, 13.5521) (-1.4682, 13.3417) (-2.673, 14.1668) knots 1 1 1 1 2 2 2 2
  line L258 (-2.673, 14.1668) -> (-2.6752, 14.1668) construction
  spline S64 degree 1 poles (-2.673, 14.1668) (-2.6752, 14.1668) knots 1 1 2 2
  arc A0 (-4.22, 14.3594) -> (-2.6752, 14.1668) centre (-3.4384, 14.3366) ccw
  line L259 (-3.4344, 13.8523) -> (-3.4987, 14.0167) construction
  line L260 (-3.4987, 14.0167) -> (-3.5922, 14.1456) construction
  spline S65 degree 2 poles (-3.4344, 13.8523) (-3.4987, 14.0167) (-3.5922, 14.1456) knots 1 1 1 2 2 2
  line L261 (-3.5922, 14.1456) -> (-3.6964, 14.271) construction
  line L262 (-3.6964, 14.271) -> (-3.6964, 14.36) construction
  spline S66 degree 2 poles (-3.5922, 14.1456) (-3.6964, 14.271) (-3.6964, 14.36) knots 1 1 1 2 2 2
  line L263 (-3.6964, 14.36) -> (-3.6964, 14.4475) construction
  line L264 (-3.6964, 14.4475) -> (-3.6376, 14.51) construction
  line L265 (-3.6376, 14.51) -> (-3.5917, 14.5737) construction
  spline S67 degree 3 poles (-3.6964, 14.36) (-3.6964, 14.4475) (-3.6376, 14.51) (-3.5917, 14.5737) knots 1 1 1 1 2 2 2 2
  line L266 (-3.5917, 14.5737) -> (-3.4976, 14.7011) construction
  line L267 (-3.4976, 14.7011) -> (-3.4344, 14.8659) construction
  spline S68 degree 2 poles (-3.5917, 14.5737) (-3.4976, 14.7011) (-3.4344, 14.8659) knots 1 1 1 2 2 2
  line L268 (-3.4344, 13.8523) -> (-3.3701, 14.0167) construction
  line L269 (-3.3701, 14.0167) -> (-3.2766, 14.1456) construction
  spline S69 degree 2 poles (-3.4344, 13.8523) (-3.3701, 14.0167) (-3.2766, 14.1456) knots 1 1 1 2 2 2
  line L270 (-3.2766, 14.1456) -> (-3.1724, 14.271) construction
  line L271 (-3.1724, 14.271) -> (-3.1724, 14.36) construction
  spline S70 degree 2 poles (-3.2766, 14.1456) (-3.1724, 14.271) (-3.1724, 14.36) knots 1 1 1 2 2 2
  line L272 (-3.1724, 14.36) -> (-3.1724, 14.4475) construction
  line L273 (-3.1724, 14.4475) -> (-3.2311, 14.51) construction
  line L274 (-3.2311, 14.51) -> (-3.277, 14.5737) construction
  spline S71 degree 3 poles (-3.1724, 14.36) (-3.1724, 14.4475) (-3.2311, 14.51) (-3.277, 14.5737) knots 1 1 1 1 2 2 2 2
  line L275 (-3.277, 14.5737) -> (-3.3711, 14.7011) construction
  line L276 (-3.3711, 14.7011) -> (-3.4344, 14.8659) construction
  spline S72 degree 2 poles (-3.277, 14.5737) (-3.3711, 14.7011) (-3.4344, 14.8659) knots 1 1 1 2 2 2
  line L277 (-43.2454, 6.7956) -> (-41.2454, 4.7956) projected
  line L278 (33.7546, -7.2044) -> (33.7546, 4.7956) projected
  line L279 (-29.7595, -18.7044) -> (22.2546, -18.7044) projected
  line L280 (-41.2454, 4.7956) -> (-41.2454, -7.2044) projected
  arc A1 (13.2546, 21.2956) -> (9.2546, 25.2956) centre (9.2546, 21.2956) ccw projected
  line L281 (-8.4354, 25.2956) -> (0.9446, 25.2956) projected
  line L282 (-5.9522, 5.3392) -> (-5.925, 5.3649)
  point P0 (0, 0)
  constraints: 5 horizontal, 5 vertical, 4 point on line, 2 end point, 2 point on circle, 1 centre point, 1 collinear, 219 other
extrude "Wyciągnięcie proste9" cut sketch "Szkic14" along normal blind 1.7 from surface at -2.5